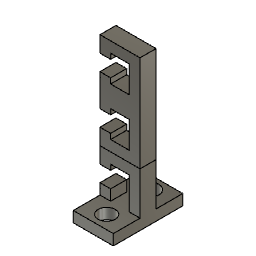
ESC_Holder_Kane_2-6-20 (Autodesk Fusion 360 archive; units mm, degrees)
design "esc holder mount"
Autodesk Fusion 360 part; units mm, degrees
note: some values were not read from the file. Chosen so that the rebuilt part matches the saved one: which bodies a step acts on.
sketch "Sketch1" plane through (0, 0, 0) normal (0, 1, 0) x (1, 0, 0)
  line L0 (0, 0) -> (-3.5, 0)
  line L1 (-3.5, 0) -> (-5.5, 0)
  line L2 (0, 0) -> (2, 0)
  line L3 (2, 0) -> (2, -4.5)
  line L4 (2, -4.5) -> (2, -9)
  line L5 (2, -9) -> (0, -9)
  line L6 (0, -9) -> (-3.5, -9)
  line L7 (-3.5, -9) -> (-5.5, -9)
  line L8 (0, 0) -> (0, -9)
  line L9 (-5.5, 0) -> (-5.5, -2)
  line L10 (-5.5, -2) -> (0, -2)
  line L11 (-5.5, -9) -> (-5.5, -7)
  line L12 (-5.5, -7) -> (0, -7)
  line L13 (-3.5089, -2) -> (-3.5089, -3)
  line L14 (-3.5089, -3) -> (-5.5089, -3)
  line L15 (-5.5089, -3) -> (-5.5, -2)
  line L16 (-5.5, -7) -> (-5.5, -6)
  line L17 (-5.5, -6) -> (-3.5, -6)
  line L18 (-3.5, -6) -> (-3.5, -7)
  dimension "d2" = 3.5
  dimension "d3" = 2
  dimension "d4" = 2
  dimension "d5" = 4.5
  dimension "d6" = 4.5
  dimension "d7" = 2
  dimension "d8" = 3.5
  dimension "d9" = 2
  dimension "d10" = 2
  dimension "d11" = 2
  dimension "d12" = 1
  dimension "d13" = 2
  dimension "d14" = 1
  dimension "d15" = 2
  constraint coincident L0.start L2.start
  constraint horizontal L0
  constraint parallel L0 L1
  constraint parallel L0 L2
  constraint perpendicular L2 L3
  constraint parallel L3 L4
  constraint perpendicular L4 L5
  constraint parallel L5 L6
  constraint parallel L6 L7
  constraint perpendicular L1 L9
  constraint coincident L8 L10.end
  constraint perpendicular L8 L10
  constraint perpendicular L7 L11
  constraint coincident L8 L12.end
  constraint perpendicular L8 L12
  constraint coincident L10 L13.start
  constraint perpendicular L10 L13
  constraint perpendicular L13 L14
  constraint perpendicular L12 L16
  constraint perpendicular L16 L17
  constraint coincident L12 L18.end
  constraint perpendicular L12 L18
  measures "d2" distance of L0.start L0.end
  measures "d3" distance of L0.end L1.end
  measures "d4" distance of L0.start L2.end
  measures "d5" distance of L2.end L3.end
  measures "d6" distance of L3.end L4.end
  measures "d7" distance of L4.end L5.end
  measures "d8" distance of L5.end L6.end
  measures "d9" distance of L6.end L7.end
  measures "d10" distance of L1.end L9.end
  measures "d11" distance of L7.end L11.end
  measures "d12" distance of L13.start L13.end
  measures "d13" distance of L13.end L14.end
  measures "d14" distance of L11.end L16.end
  measures "d15" distance of L16.end L17.end
extrude "Extrude1" add sketch "Sketch1" along normal blind 3 makes body 1
copy_body "CopyPasteBodies1" bodies 1 makes body 2
move_body "Move1" bodies 2 to x (1, 0, 0) y (0, 1, 0) z (0, 0, 1) at (0, 9, 9)
copy_body "CopyPasteBodies2" bodies 2 makes body 3
move_body "Move2" bodies 3 to x (1, 0, 0) y (0, 1, 0) z (0, 0, 1) at (0, 9, 9)
combine "Combine1" operation add target body 3 tool bodies 2 1 makes body 4 at (1.3333, 9, 14.3333) makes body 5 at (1.3333, 0, 5.3333)
move_body "Move3" bodies 4 to x (1, 0, 0) y (0, 1, 0) z (0, 0, 1) at (0, -9, 0)
move_body "Move4" bodies 3 to x (1, 0, 0) y (0, 1, 0) z (0, 0, 1) at (0, -18, 0)
sketch "Sketch2" plane through (0, 0, 0) normal (0, -1, 0) x (1, 0, 0)
  line L0 (-5.5, 0) -> (2, 0)
  line L1 (2, 0) -> (2, 9)
  line L2 (2, 9) -> (-5.5, 9)
  line L3 (-5.5, 9) -> (-5.5, 6)
  line L4 (-5.5, 6) -> (-3.5, 6)
  line L5 (-3.5, 6) -> (-3.5, 7)
  line L6 (-3.5, 7) -> (0, 7)
  line L7 (0, 7) -> (0, 2)
  line L8 (0, 2) -> (-3.5089, 2)
  line L9 (-3.5089, 2) -> (-3.5089, 3)
  line L10 (-3.5089, 3) -> (-5.5089, 3)
  line L11 (-5.5089, 3) -> (-5.5, 2)
  line L12 (-5.5, 2) -> (-5.5, 0)
  line L13 (2, 0) -> (-5.5, 0)
  line L14 (-5.5, 0) -> (-5.5, 2)
  line L15 (-5.5, 2) -> (2, 2)
  line L16 (2, 2) -> (2, 0)
  constraint horizontal L13
  constraint vertical L14
  constraint horizontal L15
  constraint vertical L16
  constraint coincident L11.end L12.start
  constraint coincident L0.end L1.start
extrude "Extrude2" add sketch "Sketch2" along normal blind 5 contours L0 L1 L8 L12 L13 L14 L15 L16 bodies 5
sketch "Sketch3" plane through (0, 0, 2) normal (0, 0, 1) x (-1, 0, 0)
  line L0 (0, 0) -> (0, -3)
  line L1 (0, -3) -> (3.5089, -3)
  line L2 (3.5089, -3) -> (3.5089, 0)
  line L3 (3.5089, 0) -> (5.5, 0)
  line L4 (5.5, 0) -> (5.5, 5)
  line L5 (5.5, 5) -> (-2, 5)
  line L6 (-2, 5) -> (-2, 0)
  line L7 (-2, 0) -> (0, 0)
  line L8 (5.5, 2.5) -> (1.75, 2.5)
  circle A0 centre (1.75, 2.5) radius 1.6
  dimension "d20" = 3.75
  dimension "d21" = 3.2
  constraint midpoint L4 L8.start
  constraint perpendicular L4 L8
  constraint coincident L8.end A0.centre
  measures "d20" distance of L8.start L8.end
  measures "d21" diameter of A0
extrude "Extrude3" cut sketch "Sketch3" against normal blind 5.5 contours A0 bodies 5
sketch "Sketch4" plane through (0, 3, 0) normal (0, 1, 0) x (-1, 0, 0)
  line L0 (-2, 0) -> (5.5, 0)
  line L1 (5.5, 0) -> (5.5, 2)
  line L2 (5.5, 2) -> (5.5089, 3)
  line L3 (5.5089, 3) -> (3.5089, 3)
  line L4 (3.5089, 3) -> (3.5089, 2)
  line L5 (3.5089, 2) -> (0, 2)
  line L6 (0, 2) -> (0, 7)
  line L7 (0, 7) -> (3.5, 7)
  line L8 (3.5, 7) -> (3.5, 6)
  line L9 (3.5, 6) -> (5.5, 6)
  line L10 (5.5, 6) -> (5.5, 9)
  line L11 (5.5, 9) -> (-2, 9)
  line L12 (-2, 9) -> (-2, 0)
  line L13 (5.5, 0) -> (-2, 0)
  line L14 (-2, 0) -> (-2, 2)
  line L15 (-2, 2) -> (5.5, 2)
  line L16 (5.5, 2) -> (5.5, 0)
  constraint horizontal L13
  constraint vertical L14
  constraint horizontal L15
  constraint vertical L16
  constraint coincident L12 L14.end
  constraint coincident L0.end L1.start
extrude "Extrude4" add sketch "Sketch4" along normal blind 5 contours L0 L1 L5 L12 L13 L14 L15 L16 bodies 5
sketch "Sketch5" plane through (0, 0, 2) normal (0, 0, 1) x (-1, 0, 0)
  circle A0 centre (1.75, 2.5) radius 1.6
  line L0 (0, 0) -> (0, -3)
  line L1 (0, -3) -> (-2, -3)
  line L2 (-2, -3) -> (-2, -8)
  line L3 (-2, -8) -> (5.5, -8)
  line L4 (5.5, -8) -> (5.5, -3)
  line L5 (5.5, -3) -> (3.5089, -3)
  line L6 (3.5089, -3) -> (3.5089, 0)
  line L7 (3.5089, 0) -> (5.5, 0)
  line L8 (5.5, 0) -> (5.5, 5)
  line L9 (5.5, 5) -> (-2, 5)
  line L10 (-2, 5) -> (-2, 0)
  line L11 (-2, 0) -> (0, 0)
  line L12 (5.5, -5.5) -> (1.75, -5.5)
  dimension "d26" = 3.75
  constraint midpoint L4 L12.start
  constraint perpendicular L4 L12
  measures "d26" distance of L12.start L12.end
sketch "Sketch6" plane through (0, 0, 2) normal (0, 0, 1) x (1, 0, 0)
  circle A0 centre (-1.75, 5.5) radius 1.75
  dimension "d27" = 3.5
  measures "d27" diameter of A0
extrude "Extrude5" cut sketch "Sketch6" against normal blind 8 bodies 5
extrude "Extrude6" cut sketch "Sketch5" against normal blind 1 bodies 5
extrude "Extrude7" add 1 faces at (-4.7756, 2.5802, 0) along direction (0, 0, -1) blind 1 on bodies 5 bodies 5
combine "Combine2" operation add target body 3 tool bodies 4
